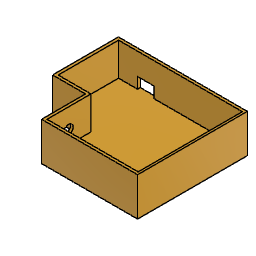
Box (Autodesk Fusion 360 design; units mm, degrees)
Autodesk Fusion 360 part; units mm, degrees
sketch "Sketch1" plane through (0, 0, 0) normal (0, 0, 1) x (1, 0, 0)
  line L0 (10, 80) -> (170, 80)
  line L1 (170, 80) -> (170, -95)
  line L2 (170, -95) -> (10, -95)
  line L3 (10, -95) -> (10, 80)
  dimension "d1" = 160
  dimension "d2" = 175
  constraint horizontal L0
  constraint vertical L1
  constraint horizontal L2
  constraint vertical L3
  measures "d1" distance of L0.start L0.end
  measures "d2" distance of L0.start L2.end
extrude "Extrude1" add sketch "Sketch1" along normal blind 90
sketch "Sketch2" plane through (0, 0, 0) normal (0, 0, 1) x (1, 0, 0)
  line L0 (10, -25, -5) -> (70, -25, -5)
  line L1 (70, -25, -5) -> (70, -95, -5)
  line L2 (70, -95, -5) -> (10, -95, -5)
  line L3 (10, -95, -5) -> (10, -25, -5)
  dimension "d5" = 60
  dimension "d6" = 70
extrude "Extrude2" cut sketch "Sketch2" along normal blind 120 contours L0 L1 L2 L3 in plane through (0, 0, -5) normal (0, 0, 1)
shell "Shell1" thickness 10 removed faces 1 at (136.6667, -13.3333, 90)
sketch "Sketch4" plane through (0, 0, 0) normal (1, 0, 0) x (0, 1, 0)
  circle A0 through (-65, 22.5, 70) (-76.25, 28.9952, 70) (-76.25, 16.0048, 70)
  circle A1 through (-40, 22.5, 70) (-51.25, 28.9952, 70) (-51.25, 16.0048, 70)
  dimension "d10" = 15
  dimension "d11" = 15
extrude "Extrude3" cut sketch "Sketch4" along normal blind 45 contours A0 | A1 in plane through (70, 0, 0) normal (1, 0, 0)
extrude "Extrude4" add 1 faces at (63.3333, 80, 30) along direction (0, 1, 0) blind 10
extrude "Extrude5" cut 1 faces at (66.6667, 70, 63.3333) along direction (0, 1, 0) blind 10
extrude "Extrude6" add 1 faces at (63.3333, 90, 30) along direction (0, 1, 0) blind 5
extrude "Extrude7" add 1 faces at (66.6667, 80, 63.3333) along direction (0, -1, 0) blind 5
extrude "Extrude8" cut 1 faces at (66.6667, 75, 63.3333) along direction (0, 1, 0) blind 10
sketch "Sketch5" plane through (0, 95, 0) normal (0, 1, 0) x (-1, 0, 0)
  line L0 (-170, 0) -> (-10, 0)
  line L1 (-10, 0) -> (-10, 90)
  line L2 (-10, 90) -> (-170, 90)
  line L3 (-170, 90) -> (-170, 0)
  line L4 (-80, 30) -> (-50, 30)
  line L5 (-50, 30) -> (-50, 10)
  line L6 (-50, 10) -> (-80, 10)
  line L7 (-80, 10) -> (-80, 30)
  constraint horizontal L4
  constraint vertical L5
  constraint horizontal L6
  constraint vertical L7
extrude "Extrude9" cut sketch "Sketch5" against normal blind 40 contours L4 L5 L6 L7
move_face "OffsetFaces1" offset -20 1 faces at (166.6667, -28.3333, 90)
move_face "MoveFace1" to x (1, 0, 0) y (0, 1, 0) z (0, 0, 1) at (-3.3857, 9.9384, -1.9072) 2 faces at (73.3333, -40.0093, 22.8738) (73.3333, -65.0093, 22.8738)
sketch "Sketch6" plane through (0, 0, 0) normal (0, 0, 1) x (1, 0, 0)
extrude "Extrude10" add 1 faces at (106.6667, -95, 46.6667) along direction (0, -1, 0) blind 10
extrude "Extrude11" cut 1 faces at (133.3333, -85, 30) along direction (0, -1, 0) blind 10
sketch "Sketch7" plane through (0, 0, 70) normal (0, 0, 1) x (-1, 0, 0)
  line L0 (-80, 95) -> (-80, 15)
  line L1 (-80, 15) -> (-20, 15)
  line L2 (-20, 15) -> (-20, -85)
  line L3 (-20, -85) -> (-160, -85)
  line L4 (-160, -85) -> (-160, 95)
  line L5 (-160, 95) -> (-80, 95)
  line L6 (-10, 25) -> (-70, 25)
  line L7 (-70, 25) -> (-70, 105)
  line L8 (-70, 105) -> (-170, 105)
  line L9 (-170, 105) -> (-170, -95)
  line L10 (-170, -95) -> (-10, -95)
  line L11 (-10, -95) -> (-10, 25)
  line L12 (-74.9369, 25) -> (-74.9369, 100)
  line L13 (-74.9369, 100) -> (-166.028, 100)
  line L14 (-166.028, 100) -> (-166.028, -90)
  line L15 (-166.028, -90) -> (-15.2566, -90)
  line L16 (-15.2566, -90) -> (-15.2566, 20)
  line L17 (-15.2566, 20) -> (-74.9369, 20)
  line L18 (-74.9369, 20) -> (-74.9369, 25)
  constraint parallel L7 L12
  constraint perpendicular L12 L13
  constraint perpendicular L10 L14
  constraint perpendicular L11 L15
  constraint perpendicular L10 L16
  constraint perpendicular L12 L17
  constraint perpendicular L17 L18
extrude "Extrude12" cut sketch "Sketch7" against normal blind 60 contours L12 L13 L14 L15 L16 L17 L18
move_face "OffsetFaces2" offset -1 1 faces at (73.2913, -30.0988, 21.3395)
move_face "MoveFace2" to x (1, 0, 0) y (0, 1, 0) z (0, 0, 1) at (1.6156, -23.2829, 13.3101) 2 faces at (71.6456, -55.0709, 20.9666) (71.6456, -29.0721, 21.0165)
move_face "OffsetFaces3" offset -1 1 faces at (73.2913, -78.3818, 34.6496)
extrude "Extrude13" add 1 faces at (170, -38.3333, 23.3333) along direction (1, 0, 0) blind 10
extrude "Extrude14" cut 1 faces at (166.028, -36.6667, 50) along direction (1, 0, 0) blind 10
extrude "Extrude15" add 1 faces at (180, -38.3333, 23.3333) along direction (1, 0, 0) blind 30
extrude "Extrude16" add 1 faces at (210, -38.3333, 23.3333) along direction (1, 0, 0) blind 5
extrude "Extrude17" cut 1 faces at (176.028, -36.6667, 50) along direction (1, 0, 0) blind 35
extrude "Extrude18" add 1 faces at (215, -38.3333, 23.3333) along direction (1, 0, 0) blind 30
extrude "Extrude19" cut 1 faces at (211.028, -36.6667, 50) along direction (1, 0, 0) blind 30
